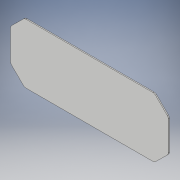
# Autodesk Inventor part: Nameplate
Saved by Autodesk Inventor 2018.3 (Build 223284000, 284)
## iProperties
Created: 2019-08-17
Part Number: Nameplate
Material: Generic
Document SubType Name: Modeling
Designer: Srinity
Density: 1 g/cm^3
Appearance: Default
Author: Srinity
Autodesk Inventor part; units mm, degrees
ref_plane "YZ Plane" through (0, 0, 0) normal (1, 0, 0) x (0, 1, 0)
ref_plane "XZ Plane" through (0, 0, 0) normal (0, 1, 0) x (-1, 0, 0)
ref_plane "XY Plane" through (0, 0, 0) normal (0, 0, 1) x (1, 0, 0)
sketch "Sketch1" plane through (0, 0, 0) normal (0, 0, 1) x (1, 0, 0)
  line L0 (-59.1185, 27.1272) -> (59.1185, 27.1272)
  line L1 (59.1185, 27.1272) -> (59.1185, 14.6685)
  line L2 (59.1185, -27.1272) -> (-59.1185, -27.1272)
  line L3 (-59.1185, -27.1272) -> (-59.1185, -14.6685)
  line L4 (-71.755, 14.6685) -> (-59.1185, 14.6685)
  line L5 (71.755, 14.6685) -> (71.755, -14.6685)
  line L6 (71.755, -14.6685) -> (59.1185, -14.6685)
  line L7 (-71.755, -14.6685) -> (-71.755, 14.6685)
  line L8 (-59.1185, 27.1272) -> (-71.755, 14.6685)
  line L9 (-71.755, -14.6685) -> (-59.1185, -27.1272)
  line L10 (59.1185, -27.1272) -> (71.755, -14.6685)
  line L11 (71.755, 14.6685) -> (59.1185, 27.1272)
  line L12 (-59.1185, 14.6685) -> (59.1185, 14.6685)
  line L13 (-59.1185, 14.6685) -> (-59.1185, 27.1272)
  line L14 (-59.1185, -14.6685) -> (-71.755, -14.6685)
  line L15 (-59.1185, -14.6685) -> (-59.1185, 14.6685)
  line L16 (59.1185, -14.6685) -> (59.1185, -27.1272)
  line L17 (59.1185, -14.6685) -> (-59.1185, -14.6685)
  line L18 (59.1185, 14.6685) -> (71.755, 14.6685)
  line L19 (59.1185, 14.6685) -> (59.1185, -14.6685)
  point P0 (0, 0)
  dimension "d0" = 118.237
  dimension "d1" = 54.2544
  dimension "d2" = 143.51
  dimension "d3" = 29.337
  dimension "d4" = 27.1272
  dimension "d5" = 59.1185
  dimension "d6" = 14.6685
  dimension "d7" = 71.755
  constraints: 40 end point, 20 parallel, 6 perpendicular, 4 horizontal
  measures "d0" distance of L0.start L0.end
  measures "d1" distance of L2.end L0.start
  measures "d2" distance of L4.start L5.start
  measures "d3" distance of L7.start L4.start
  measures "d4" distance from line of point (0, 0) L0
  measures "d5" distance from line of point (0, 0) L3
  measures "d6" distance from line of point (0, 0) L4
  measures "d7" distance from line of point (0, 0) L7
extrude "Extrusion1" add sketch "Sketch1" along normal blind 1
fillet "Fillet1" radius 3.175 8 edges at (59.1185, 27.1272, 0.5) (71.755, 14.6685, 0.5) (71.755, -14.6685, 0.5) (59.1185, -27.1272, 0.5) (-59.1185, -27.1272, 0.5) (-71.755, -14.6685, 0.5) (-71.755, 14.6685, 0.5) (-59.1185, 27.1272, 0.5)
equation "\"d4\" = 0.5 * d1"
equation "\"d5\" = 0.5 * d0"
equation "\"d6\" = 0.5 * d3"
equation "\"d7\" = 0.5 * d2"
body "Solid1"
